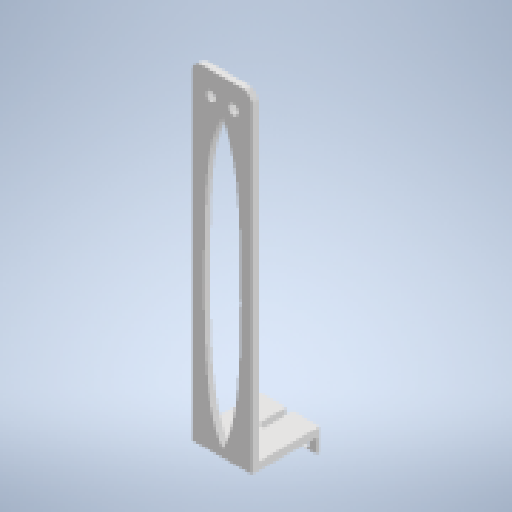
# Autodesk Inventor part: Straight_Distance_Sensor_hold
Saved by Autodesk Inventor 2023.1 (Build 271208000, 208)
## iProperties
Created: 2022-12-02
Part Number: Straight_Distance_Sensor_hold
Material: Default New Material
Document SubType Name: Modeling
Designer: Windows10
Density: 1 g/cm^3
Appearance: Generic
Author: Windows10
Autodesk Inventor part; units mm, degrees
ref_plane "YZ Plane" through (0, 0, 0) normal (1, 0, 0) x (0, 1, 0)
ref_plane "XZ Plane" through (0, 0, 0) normal (0, 1, 0) x (-1, 0, 0)
ref_plane "XY Plane" through (0, 0, 0) normal (0, 0, 1) x (1, 0, 0)
sketch "Sketch1" plane through (0, 0, 0) normal (0, 0, 1) x (1, 0, 0)
  line L0 (0, 0) -> (18.64, 0)
  line L1 (18.64, 0) -> (18.64, -7)
  line L2 (18.64, -7) -> (0, -7)
  line L3 (0, -7) -> (0, 0)
  circle A0 centre (3.95, -5.19) radius 1.75
  line L4 (9.32, 0) -> (9.32, 1.7268)
  line L5 (9.32, 0) -> (8.32, 0)
  line L6 (8.32, 0) -> (8.32, -6.4)
  line L7 (8.32, -6.4) -> (9.32, -6.4)
  line L8 (9.32, -6.4) -> (9.32, 0)
  circle A1 centre (14.69, -5.19) radius 1.75
  line L9 (10.32, 0) -> (10.32, -6.4)
  line L10 (10.32, -6.4) -> (9.32, -6.4)
  point P0 (8.82, -6.4)
  dimension "d0" = 18.64
  dimension "d1" = 7
  dimension "d2" = 5.19
  dimension "d3" = 3.5
  dimension "d4" = 3.95
  dimension "d5" = 0.6
  dimension "d6" = 1
  constraints: 22 end point, 4 parallel, 3 symmetric about line, 2 centre point, 2 horizontal, 2 midpoint, 2 perpendicular, 1 vertical, 1 other
  measures "d0" distance of L1.end L2.end
  measures "d1" distance of L0.end L1.end
  measures "d2" distance from line of L0 A0.centre
  measures "d3" diameter of A0
  measures "d4" distance from line of L3 A0.centre
  measures "d5" distance from line of L2 point (8.82, -6.4)
  measures "d6" distance of L6.end L7.end
extrude "Extrusion1" add sketch "Sketch1" along normal blind 1 contours L0 L6 L7 L10 L9 L1 L2 L3
sketch "Sketch2" plane through (0, 0, 1) normal (0, 0, 1) x (1, 0, 0)
  line L0 (0, -7) -> (18.64, -7) projected
  line L1 (18.64, -7) -> (18.64, 0) projected
  line L2 (18.64, 0) -> (10.32, 0) projected
  line L3 (10.32, -6.4) -> (8.32, -6.4) projected
  line L4 (8.32, -6.4) -> (8.32, 0) projected
  line L5 (8.32, 0) -> (0, 0) projected
  line L6 (0, 0) -> (0, -7) projected
  circle A0 centre (3.95, -5.19) radius 1.75 projected
  circle A1 centre (14.69, -5.19) radius 1.75 projected
  line L7 (8.32, 0) -> (0, 0) projected
  line L8 (8.32, -6.4) -> (8.32, 0) projected
  line L9 (0, 0) -> (8.32, 0)
  line L10 (8.32, 0) -> (8.32, -2.5)
  line L11 (8.32, -2.5) -> (0, -2.5)
  line L12 (0, -2.5) -> (0, 0)
  line L13 (9.32, 0) -> (9.32, -6.4) projected
  line L14 (18.64, -7) -> (18.64, 0) projected
  line L15 (9.32, 0) -> (18.64, 0)
  line L16 (18.64, 0) -> (18.64, -2.5)
  line L17 (18.64, -2.5) -> (9.32, -2.5)
  line L18 (9.32, -2.5) -> (9.32, 0)
  line L19 (10.32, 0) -> (10.32, -6.4) projected
  point P0 (0, -2.5)
  point P1 (10.32, -2.5)
  dimension "d9" = 2.5
  dimension "d10" = 2.5
  constraints: 16 end point, 4 parallel, 2 horizontal, 2 perpendicular, 2 point on line
  measures "d9" distance between parallel lines of L9 L11
  measures "d10" distance of L15.end L16.end
extrude "Extrusion2" add sketch "Sketch2" along normal blind 18 contours L6 L5 L4 L11 | L17 L19 L2 L1
sketch "Sketch3" plane through (8.32, -6.4, 0) normal (1, 0, 0) x (0, 0, -1)
  line L0 (0, 0) -> (0, 6.4) projected
  line L1 (0, 6.4) -> (-19, 6.4) projected
  line L2 (-19, 3.9) -> (-19, 6.4) projected
  line L3 (-1, 3.9) -> (-19, 3.9) projected
  line L4 (-1, 0) -> (-1, 3.9) projected
  line L5 (0, 0) -> (-1, 0) projected
  line L6 (-1, 3.9) -> (-19, 3.9) projected
  line L7 (-19, 6.4) -> (-9, 6.4)
  line L8 (-9, 6.4) -> (-9, 3.9)
  line L9 (-9, 3.9) -> (-19, 3.9)
  line L10 (-19, 3.9) -> (-19, 6.4)
  point P0 (0, 6.4)
  dimension "d13" = 10
  constraints: 8 end point, 2 parallel, 1 horizontal, 1 perpendicular, 1 point on line
  measures "d13" distance of L8.end L9.end
extrude "Extrusion3" add sketch "Sketch3" along normal blind 2 contours L8 L3 L2 L1
sketch "Sketch4" plane through (0, 0, 19) normal (0, 0, 1) x (1, 0, 0)
  line L0 (18.64, 0) -> (10.32, 0) projected
  line L1 (18.64, 0) -> (0, 0)
  line L2 (0, 0) -> (0, 100)
  line L3 (0, 100) -> (18.64, 100)
  line L4 (18.64, 100) -> (18.64, 0)
  line L5 (10.32, -2.5) -> (10.32, 0) projected
  line L6 (18.64, 0) -> (0, 0) projected
  line L7 (0, 0) -> (0, -2.5) projected
  line L8 (0, -2.5) -> (18.64, -2.5) projected
  line L9 (18.64, -2.5) -> (18.64, 0) projected
  dimension "d16" = 100
  constraints: 8 end point, 2 parallel, 1 horizontal, 1 perpendicular
  measures "d16" distance of L1.end L2.end
extrude "Extrusion4" add sketch "Sketch4" along normal blind 2
sketch "Sketch5" plane through (0, 0, 21) normal (0, 0, 1) x (1, 0, 0)
  circle A0 centre (12.82, 93) radius 1.5
  circle A1 centre (5.82, 93) radius 1.5
  line L0 (12.82, 93) -> (5.82, 93)
  line L1 (18.64, 100) -> (0, 100) projected
  line L2 (9.32, 100) -> (9.32, 93)
  point P0 (0, 0)
  dimension "d19" = 3
  dimension "d20" = 3
  dimension "d21" = 7
  dimension "d22" = 7
  constraints: 4 end point, 2 centre point, 2 midpoint, 1 horizontal, 1 vertical
  measures "d19" diameter of A0
  measures "d20" diameter of A1
  measures "d21" distance of L0.end L0.start
  measures "d22" distance of L2.start L2.end
extrude "Extrusion5" cut sketch "Sketch5" against normal blind 13.75
sketch "Sketch6" plane through (0, 0, 21) normal (0, 0, 1) x (1, 0, 0)
  line L0 (18.64, 100) -> (0, 100) projected
  line L1 (9.32, 100) -> (9.32, -19)
  line L2 (9.32, 89) -> (13, 82) construction
  line L3 (13, 82) -> (15, 69) construction
  line L4 (15, 69) -> (15, 40.5) construction
  line L5 (15, 40.5) -> (15, 17) construction
  line L6 (15, 17) -> (12, 4) construction
  line L7 (8.32, 0) -> (10.32, 0) projected
  line L8 (12, 4) -> (9.32, 0) construction
  spline S0 degree 4 poles (9.32, 89) (13, 82) (15, 69) (15, 40.5) (15, 17) (12, 4) (9.32, 0) knots 1 1 1 1 1 2 3 4 4 4 4 4
  line L9 (9.32, 89) -> (5.64, 82) construction
  line L10 (5.64, 82) -> (3.64, 69) construction
  line L11 (3.64, 69) -> (3.64, 40.5) construction
  line L12 (3.64, 40.5) -> (3.64, 17) construction
  line L13 (3.64, 17) -> (6.64, 4) construction
  line L14 (6.64, 4) -> (9.32, 0) construction
  spline S1 degree 4 poles (9.32, 89) (5.64, 82) (3.64, 69) (3.64, 40.5) (3.64, 17) (6.64, 4) (9.32, 0) knots 1 1 1 1 1 2 3 4 4 4 4 4
  point P0 (0, 0)
  constraints: 5 symmetric about line, 3 vertical, 2 end point, 2 midpoint, 1 point on line, 6 other
extrude "Extrusion6" cut sketch "Sketch6" against normal blind 13.75
fillet "Fillet1" radius 3 2 edges at (0, 100, 20) (18.64, 100, 20)
body "Solid1"
